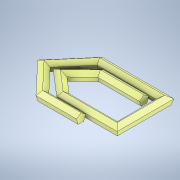
# Autodesk Inventor part: Pin
Saved by Autodesk Inventor 2021 (Build 250183000, 183)
## iProperties
Created: 2021-07-28
Part Number: Pin
Material: Generic
Document SubType Name: Modeling
Designer: Shammy Haider
Density: 1 g/cm^3
Appearance: Default
Author: Shammy Haider
Autodesk Inventor part; units mm, degrees
ref_plane "YZ Plane" through (0, 0, 0) normal (1, 0, 0) x (0, 1, 0)
ref_plane "XZ Plane" through (0, 0, 0) normal (0, 1, 0) x (-1, 0, 0)
sketch "Sketch1" plane through (0, 0, 0) normal (0, 1, 0) x (-1, 0, 0)
  line L0 (1.944, 6.2906) -> (10.8557, 6.2906)
  line L1 (10.8557, 6.2906) -> (16.7968, 0)
  line L2 (16.7968, 0) -> (10.8557, -6.9022)
  line L3 (10.8557, -6.9022) -> (-4.2156, -6.9022)
  line L4 (-4.2156, -6.9022) -> (-4.2156, 4.1064)
  line L5 (-4.2156, 4.1064) -> (8.313, 4.1064)
  line L6 (8.313, 4.1064) -> (13.0836, 0)
  line L7 (13.0836, 0) -> (8.313, -4.5869)
  line L8 (8.313, -4.5869) -> (-1.7256, -4.5869)
  point P0 (0, 0)
  constraints: 18 end point, 3 perpendicular, 2 parallel, 1 horizontal
ref_plane "Work Plane1" through (-1.944, 0, 6.2906) normal (-1, 0, 0) x (0, -1, 0)
sketch "Sketch2" plane through (-1.944, 0, 6.2906) normal (-1, 0, 0) x (0, -1, 0)
  line L0 (0.9091, -0.605) -> (-0.2945, -1.0515)
  line L1 (-0.2945, -1.0515) -> (-1.0911, -0.0449)
  line L2 (-1.0911, -0.0449) -> (-0.3798, 1.0238)
  line L3 (-0.3798, 1.0238) -> (0.8563, 0.6776)
  line L4 (0.8563, 0.6776) -> (0.9091, -0.605)
  point P0 (0, -6.2906)
  point P1 (0, 0)
  dimension "d2" = 2.0753
  constraints: 10 end point, 11 other
  measures "d2" vertical distance of L2.end L0.end
sweep "Sweep1" add profiles "Sketch2" path "Sketch1"
body "Solid1"
